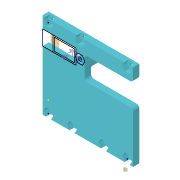
# Autodesk Inventor part: SensorWall
Saved by Autodesk Inventor 2018 (Build 220112000, 112)
## iProperties
Created: 2018-12-09
Part Number: SensorWall
Material: Generic
Document SubType Name: Modeling
Designer: ball
Density: 1 g/cm^3
Appearance: Default
Author: ball
Autodesk Inventor part; units mm, degrees
ref_plane "YZ Plane" through (0, 0, 0) normal (1, 0, 0) x (0, 1, 0)
ref_plane "XZ Plane" through (0, 0, 0) normal (0, 1, 0) x (-1, 0, 0)
ref_plane "Work Plane1" through (0, 0, 0) normal (0, 0, 1) x (1, 0, 0)
sketch "Sketch1" plane through (0, 0, 0) normal (0, 0, 1) x (1, 0, 0)
  line L0 (86, -8) -> (86, -12) construction
  line L1 (116, -16) -> (-164, -16) construction
  line L2 (116, 72) -> (-164, 72) construction
  line L3 (-6, 68) -> (-6, 64) construction
  line L4 (86, -16) -> (-6, -16)
  line L5 (-6, -16) -> (-6, 71.503)
  line L6 (-6, 71.503) -> (36.75, 71.503)
  line L7 (86, 35.181) -> (86, -16)
  line L8 (58.1676, 40.25) -> (85.5305, 40.25) construction
  line L9 (36.75, 47.9255) -> (36.75, 56.0811) construction
  line L10 (86, 35.181) -> (36.75, 35.181)
  line L11 (36.75, 35.181) -> (36.75, 58.041)
  line L12 (36.75, 71.503) -> (86, 71.503)
  line L13 (86, 71.503) -> (86, 58.041)
  line L14 (86, 58.041) -> (36.75, 58.041)
  point P0 (0, 0)
  dimension "d0" = 87.503
  dimension "d71" = 13.462
  constraints: 30 end point, 5 horizontal, 3 parallel, 3 vertical, 2 perpendicular, 2 point on line, 12 other
  measures "d0" distance of L4.end L5.end
  measures "d71" distance of L12.end L13.end
extrude "Extrusion1" add sketch "Sketch1" along normal blind 6.35
sketch "Sketch3" plane through (0, 0, 6.35) normal (0, 0, 1) x (1, 0, 0)
  circle A0 centre (32, 68) radius 2 construction
  point P0 (0, 0)
  constraints: 1 centre point, 2 other
hole "Hole2" at (32, 68, 6.35) direction (0, 0, -1) diameter 3.9878 end through all
sketch "Sketch4" plane through (0, 0, 6.35) normal (0, 0, 1) x (1, 0, 0)
  circle A0 centre (80, -12) radius 2 construction
  circle A1 centre (80, -12) radius 4.8768 construction
  circle A2 centre (0, -12) radius 2 construction
  circle A3 centre (0, 68) radius 2 construction
  circle A4 centre (32, 68) radius 2 construction
  circle A5 centre (0, -12) radius 4.8768 construction
  circle A6 centre (0, 68) radius 1.9939 construction
  circle A7 centre (0, 68) radius 4.8768 construction
  circle A8 centre (32, 68) radius 1.9939 construction
  circle A9 centre (32, 68) radius 4.8768 construction
  circle A10 centre (24, -12) radius 2 construction
  circle A11 centre (56, -12) radius 2 construction
  circle A12 centre (56, -12) radius 4.8768 construction
  circle A13 centre (24, -12) radius 4.8768 construction
  circle A14 centre (80, -12) radius 1.9939 projected
  line L0 (75.1232, -12) -> (77.5616, -7.7766)
  line L1 (77.5616, -7.7766) -> (82.4384, -7.7766)
  line L2 (82.4384, -7.7766) -> (84.8768, -12)
  line L3 (84.8768, -12) -> (82.4384, -16.2234)
  line L4 (82.4384, -16.2234) -> (77.5616, -16.2234)
  line L5 (77.5616, -16.2234) -> (75.1232, -12)
  line L6 (51.1232, -12) -> (53.5616, -7.7766)
  line L7 (53.5616, -7.7766) -> (58.4384, -7.7766)
  line L8 (58.4384, -7.7766) -> (60.8768, -12)
  line L9 (60.8768, -12) -> (58.4384, -16.2234)
  line L10 (58.4384, -16.2234) -> (53.5616, -16.2234)
  line L11 (53.5616, -16.2234) -> (51.1232, -12)
  line L12 (19.1232, -12) -> (21.5616, -7.7766)
  line L13 (21.5616, -7.7766) -> (26.4384, -7.7766)
  line L14 (26.4384, -7.7766) -> (28.8768, -12)
  line L15 (28.8768, -12) -> (26.4384, -16.2234)
  line L16 (26.4384, -16.2234) -> (21.5616, -16.2234)
  line L17 (21.5616, -16.2234) -> (19.1232, -12)
  line L18 (-4.8768, -12) -> (-2.4384, -7.7766)
  line L19 (-2.4384, -7.7766) -> (2.4384, -7.7766)
  line L20 (2.4384, -7.7766) -> (4.8768, -12)
  line L21 (4.8768, -12) -> (2.4384, -16.2234)
  line L22 (2.4384, -16.2234) -> (-2.4384, -16.2234)
  line L23 (-2.4384, -16.2234) -> (-4.8768, -12)
  line L24 (27.1232, 68) -> (29.5616, 72.2234)
  line L25 (29.5616, 72.2234) -> (34.4384, 72.2234)
  line L26 (34.4384, 72.2234) -> (36.8768, 68)
  line L27 (36.8768, 68) -> (34.4384, 63.7766)
  line L28 (34.4384, 63.7766) -> (29.5616, 63.7766)
  line L29 (29.5616, 63.7766) -> (27.1232, 68)
  line L30 (-4.8768, 68) -> (-2.4384, 72.2234)
  line L31 (-2.4384, 72.2234) -> (2.4384, 72.2234)
  line L32 (2.4384, 72.2234) -> (4.8768, 68)
  line L33 (4.8768, 68) -> (2.4384, 63.7766)
  line L34 (2.4384, 63.7766) -> (-2.4384, 63.7766)
  line L35 (-2.4384, 63.7766) -> (-4.8768, 68)
  point P0 (0, 0)
  dimension "d18" = 9.7536
  dimension "d21" = 9.7536
  dimension "d22" = 9.7536
  dimension "d23" = 9.7536
  dimension "d24" = 9.7536
  dimension "d25" = 9.7536
  constraints: 72 end point, 12 coincident, 6 centre point, 6 horizontal alignment, 102 other
extrude "Extrusion2" cut sketch "Sketch4" against normal blind 4.6228
sketch "Sketch5" plane through (0, 0, 6.35) normal (0, 0, 1) x (1, 0, 0)
  circle A0 centre (56, -12) radius 2 construction
  circle A1 centre (24, -12) radius 2 construction
  point P0 (0, 0)
  constraints: 2 centre point, 4 other
hole "Hole3" at (56, -12, 6.35) at (24, -12, 6.35) direction (0, 0, -1) diameter 3.9878 end through all
sketch "Sketch6" plane through (0, 0, 6.35) normal (0, 0, 1) x (1, 0, 0)
  circle A0 centre (32, 52) radius 1.8 construction
  line L0 (25.6709, 58.1897) -> (15.8763, 58.1897) construction
  line L1 (15.8763, 45.8103) -> (25.6716, 45.8103) construction
  line L2 (26.268, 46.528) -> (26.268, 49.5214) construction
  line L3 (5.9638, 51.1237) -> (5.9638, 48.0771) construction
  circle A1 centre (32, 52) radius 1.778
  circle A2 centre (32, 52) radius 4.8768 construction
  line L4 (27.1232, 52) -> (29.5616, 56.2234)
  line L5 (29.5616, 56.2234) -> (34.4384, 56.2234)
  line L6 (34.4384, 56.2234) -> (36.8768, 52)
  line L7 (36.8768, 52) -> (34.4384, 47.7766)
  line L8 (34.4384, 47.7766) -> (29.5616, 47.7766)
  line L9 (29.5616, 47.7766) -> (27.1232, 52)
  line L10 (26.268, 45.875) -> (5.9638, 45.875)
  line L11 (5.9638, 45.875) -> (5.9638, 58.1897)
  line L12 (5.9638, 58.1897) -> (26.268, 58.1897)
  line L13 (26.268, 58.1897) -> (26.268, 45.875)
  line L14 (4.5388, 44.45) -> (27.693, 44.45)
  line L15 (27.693, 44.45) -> (27.693, 59.6147)
  line L16 (27.693, 59.6147) -> (4.5388, 59.6147)
  line L17 (4.5388, 59.6147) -> (4.5388, 44.45)
  line L18 (27.693, 44.45) -> (4.5388, 44.45)
  line L19 (4.5388, 44.45) -> (4.5388, 59.6147)
  line L20 (4.5388, 59.6147) -> (27.693, 59.6147)
  line L21 (27.693, 59.6147) -> (27.693, 44.45)
  line L22 (-6, 71.503) -> (-6, -16) construction
  line L23 (4.5388, 59.6147) -> (-6, 59.6147)
  line L24 (-6, 59.6147) -> (-6, 44.45)
  line L25 (-6, 44.45) -> (4.5388, 44.45)
  line L26 (4.5388, 44.45) -> (4.5388, 59.6147)
  circle A3 centre (0, -12) radius 2 construction
  circle A4 centre (0, 68) radius 2 construction
  circle A5 centre (80, -12) radius 2 construction
  point P0 (0, 0)
  dimension "d36" = 9.7536
  dimension "d35" = 3.556
  dimension "d48" = 1.425
  constraints: 52 end point, 8 parallel, 5 centre point, 5 horizontal, 4 perpendicular, 3 coincident, 2 vertical, 1 horizontal alignment, 1 point on line, 34 other
  measures "d35" diameter of A1
  measures "d48" distance between parallel lines of L10 L14
hole "Hole4" at (32, 52, 6.35) direction (0, 0, -1) diameter 3.556 end through all
extrude "Extrusion3" cut sketch "Sketch6" against normal blind 4.6228 contours L4 L15 L9 | L4 L5 L6 L7 L8 L9 L15
extrude "Extrusion4" cut sketch "Sketch6" against normal through all contours L10 L11 L12 L13
extrude "Extrusion5" cut sketch "Sketch6" against normal through all contours L9 L15 L14 L17 L16 L4 | L4 L15 L9
sketch "Sketch7" plane through (0, 0, 0) normal (0, 0, -1) x (-1, 0, 0)
  line L0 (-27.693, 59.6147) -> (-4.5388, 59.6147) projected
  line L1 (-4.5388, 59.6147) -> (-4.5388, 44.45) projected
  line L2 (-4.5388, 44.45) -> (-27.693, 44.45) projected
  line L3 (-27.693, 44.45) -> (-27.693, 59.6147) projected
  circle A0 centre (-32, 52) radius 1.778 projected
  circle A1 centre (-56, -12) radius 1.9939 projected
  circle A2 centre (-24, -12) radius 1.9939 projected
  circle A3 centre (-32, 68) radius 1.9939 projected
  line L4 (-86, -16) -> (6, -16) projected
  line L5 (6, -16) -> (6, 71.503) projected
  line L6 (6, 71.503) -> (-86, 71.503) projected
  line L7 (-36.75, 58.041) -> (-36.75, 35.181) projected
  line L8 (-36.75, 35.181) -> (-86, 35.181) projected
  line L9 (-86, 35.181) -> (-86, -16) projected
  line L10 (1.3245, 44.5) -> (-33.3311, 44.5) construction
  line L11 (-33.3245, 59.5) -> (1.3311, 59.5) construction
  line L12 (-27.693, 44.45) -> (-27.693, 59.6147) construction
  line L13 (-27.693, 44.45) -> (-4.5388, 44.45) projected
  line L14 (-36.75, 52.2196) -> (-36.75, 58.041) projected
  line L15 (-27.693, 44.45) -> (-36.75, 44.45)
  line L16 (-36.75, 44.45) -> (-36.75, 59.6147)
  line L17 (-36.75, 59.6147) -> (-27.693, 59.6147)
  line L18 (-27.693, 59.6147) -> (-27.693, 44.45)
  line L19 (-86, 71.503) -> (-86, 58.041) projected
  line L20 (-86, 58.041) -> (-36.75, 58.041) projected
  point P0 (0, 0)
  point P1 (-36.75, 67.7804)
  constraints: 12 end point, 3 horizontal, 2 parallel, 1 perpendicular, 1 point on line, 4 other
ref_plane "Work Plane2" through (27.2145, 45.1271, -7.45) normal (0, 0, 1) x (1, 0, 0)
extrude "Extrusion6" add sketch "Sketch7" along normal up to surface (7.45 mm away) contours L3 L15 L7 L16 L17
sketch "Sketch8" plane through (-6, -16, 0) normal (-1, 0, 0) x (0, 0, 1)
  point P0 (0, 16)
extrude "Extrusion7" cut sketch "Sketch6" against normal through all contours L17 L25 L24 L23
hole "Hole5" at (80, -12, 6.35) at (0, -12, 6.35) at (0, 68, 6.35) direction (0, 0, -1) diameter 3.556 end through all
fillet "Fillet1" radius 1.524 1 edges at (32.2215, 44.45, 0)
fillet "Fillet2" radius 3.175 3 edges at (32.2215, 59.6147, 0) (36.75, 35.181, 3.175) (86, 35.181, 3.175)
hole "Hole6" at (80, -12, 6.35) direction (0, 0, -1) diameter 3.9878 end through all
fillet "Fillet3" radius 3.175 1 edges at (86, 58.041, 3.175)
fillet "Fillet4" radius 3.175 1 edges at (36.75, 58.041, 3.175)
sketch "Sketch9" plane through (0, 0, 6.35) normal (0, 0, 1) x (1, 0, 0)
  circle A0 centre (80, 68) radius 2 construction
  circle A1 centre (80, 68) radius 4.8768 construction
  line L0 (75.1232, 68) -> (77.5616, 72.2234)
  line L1 (77.5616, 72.2234) -> (82.4384, 72.2234)
  line L2 (82.4384, 72.2234) -> (84.8768, 68)
  line L3 (84.8768, 68) -> (82.4384, 63.7766)
  line L4 (82.4384, 63.7766) -> (77.5616, 63.7766)
  line L5 (77.5616, 63.7766) -> (75.1232, 68)
  circle A2 centre (80, 68) radius 1.9939
  point P0 (0, 0)
  dimension "d74" = 9.7536
  dimension "d75" = 3.9878
  constraints: 12 end point, 3 coincident, 2 centre point, 1 horizontal alignment, 17 other
  measures "d75" diameter of A2
extrude "Extrusion8" cut sketch "Sketch9" against normal through all contours A2
sketch "Sketch10" plane through (0, 0, 6.35) normal (0, 0, 1) x (1, 0, 0)
  circle A0 centre (80, 68) radius 1.9939 construction
  circle A1 centre (80, 68) radius 4.8768 construction
  line L0 (75.1232, 68) -> (77.5616, 72.2234)
  line L1 (77.5616, 72.2234) -> (82.4384, 72.2234)
  line L2 (82.4384, 72.2234) -> (84.8768, 68)
  line L3 (84.8768, 68) -> (82.4384, 63.7766)
  line L4 (82.4384, 63.7766) -> (77.5616, 63.7766)
  line L5 (77.5616, 63.7766) -> (75.1232, 68)
  point P0 (0, 0)
  dimension "d78" = 9.7536
  constraints: 12 end point, 2 coincident, 1 horizontal alignment, 15 other
extrude "Extrusion9" cut sketch "Sketch10" against normal blind 4.6228
body "Solid1"
